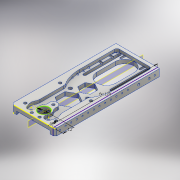
# Autodesk Inventor part: Z-head-baseplate-IKO
Saved by Autodesk Inventor 2016 (Build 200138000, 138)
## iProperties
Created: 2015-05-08
Part Number: Z-head-baseplate-IKO
Material: Aluminum 6061
Document SubType Name: Modeling
Designer: ax
Density: 2.7 g/cm^3
Appearance: Aluminum - Flat
Mass: 63.125 g
Surface Area: 166.822 cm^2
Volume: 23.3796 cm^3
Author: ax
Autodesk Inventor part; units mm, degrees
ref_plane "YZ Plane" through (0, 0, 0) normal (1, 0, 0) x (0, 1, 0)
ref_plane "XZ Plane" through (0, 0, 0) normal (0, 1, 0) x (-1, 0, 0)
ref_plane "XY Plane" through (0, 0, 0) normal (0, 0, 1) x (1, 0, 0)
sketch "Sketch1" plane through (0, 0, 0) normal (0, 0, 1) x (1, 0, 0)
  line L0 (0, 0) -> (45, 0)
  line L1 (45, 0) -> (45, 120)
  line L2 (45, 120) -> (0, 120)
  line L3 (0, 120) -> (0, 0)
  dimension "width" = 45
  dimension "height" = 120
  constraints: 8 end point, 2 parallel, 1 horizontal, 1 perpendicular
  measures "width" distance of L2.end L1.end
  measures "height" distance of L1.end L0.end
extrude "Extrusion1" add sketch "Sketch1" along normal blind 8
sketch "Sketch2" plane through (45, 0, 0) normal (1, 0, 0) x (0, 0, -1)
  line L0 (0, 0) -> (0, 120) projected
  line L1 (-8, 0) -> (-8, 120) projected
  line L2 (0, 0) -> (-8, 0)
  line L3 (-8, 0) -> (-8, 120)
  line L4 (-8, 120) -> (0, 120)
  line L5 (0, 120) -> (0, 0)
  line L6 (0, 0) -> (-8, 0) projected
  dimension "d4" = 120
  dimension "d5" = 0
  constraints: 8 end point, 2 parallel, 2 point on line, 1 horizontal, 1 perpendicular
  measures "d4" distance of L2.end L3.end
  measures "d5" distance between parallel lines of L6 L2
extrude "Extrusion2" add sketch "Sketch2" along normal blind 2.5
sketch "Sketch5" plane through (47.5, 0, 0) normal (1, 0, 0) x (0, 0, -1)
  line L0 (0, 0) -> (0, 120)
  line L1 (-8, 120) -> (-8, 0)
  line L2 (-8, 0) -> (0, 0) projected
  point P0 (-5, 12)
  point P1 (-5, 18.5)
  dimension "d11" = 6.5
  dimension "d128" = 3
  dimension "d129" = 12
  constraints: 4 end point, 1 parallel, 1 vertical
  measures "d11" distance of point (-5, 12) point (-5, 18.5)
  measures "d128" distance from line of L1 point (-5, 12)
  measures "d129" distance from line of L2 point (-5, 12)
hole "Hole1" at (47.5, 18.5, 5) at (47.5, 12, 5) direction (-1, 0, 0) diameter 1.567 depth 6.3 tip angle 118 thread size "M2x0.4" class "6H" standard "ISO Metric profile"
ref_plane "Midplane Mirror" through (22.5, 0, 0) normal (-1, 0, 0) x (0, 0, 1)
sketch "Sketch8" plane through (0, 0, 0) normal (0, 0, -1) x (-1, 0, 0)
  line L0 (-7, 116) -> (-7, 73) construction
  line L1 (-8.6, 114.4) -> (-8.6, 74.6)
  line L2 (-5.4, 74.6) -> (-5.4, 114.4)
  arc A0 (-5.4, 114.4) -> (-8.6, 114.4) centre (-7, 114.4) ccw
  arc A1 (-8.6, 74.6) -> (-5.4, 74.6) centre (-7, 74.6) ccw
  line L3 (-22.5, 120) -> (-22.5, 40) construction
  point P0 (0, 0)
  point P1 (-7, 94.5)
  dimension "d40" = 43
  dimension "d41" = 3.2
  dimension "d42" = 80
  dimension "d43" = 15.5
  constraints: 10 end point, 6 point on circle, 4 tangent, 2 centre point, 2 point on line, 2 vertical, 1 midpoint, 1 parallel
  measures "d40" distance of L0.start L0.end
  measures "d41" diameter of A1
  measures "d42" distance of L3.start L3.end
  measures "d43" distance from line of L3 point (-7, 94.5)
extrude "Extrusion3" cut sketch "Sketch8" against normal through all
sketch "Sketch9" plane through (0, 0, 8) normal (0, 0, 1) x (1, 0, 0)
  line L0 (22.5, 116) -> (22.5, 73) construction
  line L1 (11.5, 105) -> (11.5, 84)
  line L2 (33.5, 84) -> (33.5, 105)
  arc A0 (33.5, 105) -> (11.5, 105) centre (22.5, 105) ccw
  arc A1 (11.5, 84) -> (33.5, 84) centre (22.5, 84) ccw
  line L3 (0, 120) -> (0, 0) projected
  line L4 (0, 120) -> (47.5, 120) projected
  point P0 (22.5, 94.5)
  point P1 (45, 83)
  dimension "d47" = 43
  dimension "d48" = 22
  dimension "d130" = 15
  dimension "d131" = 22.5
  constraints: 8 end point, 6 point on circle, 4 tangent, 2 centre point, 2 point on line, 1 midpoint, 1 parallel, 1 vertical
  measures "d47" distance of L0.start L0.end
  measures "d48" diameter of A1
  measures "d130" distance from line of L4 A0.centre
  measures "d131" distance from line of L3 A0.centre
extrude "Extrusion4" cut sketch "Sketch9" against normal through all
sketch "Sketch10" plane through (0, 0, 0) normal (0, 0, -1) x (-1, 0, 0)
  point P0 (0, 0)
sketch "Sketch11" plane through (0, 0, 8) normal (0, 0, 1) x (1, 0, 0)
  point P0 (12.5, 52.5)
  point P1 (12.5, 7.5)
  point P2 (32.5, 52.5)
  point P3 (32.5, 7.5)
hole "Hole6" at (12.5, 52.5, 8) at (12.5, 7.5, 8) at (32.5, 52.5, 8) at (32.5, 7.5, 8) direction (0, 0, -1) diameter 4 depth 8 counterbore diameter 8 counterbore depth 3.5
sketch "Sketch13" plane through (0, 0, 8) normal (0, 0, 1) x (1, 0, 0)
  circle A0 centre (12.5, 7.5) radius 4 construction
  line L0 (12.5, 11.5) -> (32.5, 11.5) construction
  arc A1 (36.5, 7.5) -> (36.5, 7.5) centre (32.5, 7.5) ccw construction
  circle A2 centre (22.5, 12) radius 6
  circle A3 centre (22.5, 12) radius 6.55 construction
  line L1 (0, 0) -> (47.5, 0) projected
  dimension "d70" = 12
  dimension "d72" = 13.1
  dimension "d132" = 12
  constraints: 2 centre point, 2 end point, 1 coincident, 1 point on circle, 1 tangent, 1 vertical alignment, 1 other
  measures "d70" diameter of A2
  measures "d72" diameter of A3
  measures "d132" distance from line of L1 A2.centre
extrude "Extrusion5" cut sketch "Sketch13" against normal blind 4
sketch "Sketch14" plane through (22.5, 12, 4) normal (0, 0, 1) x (1, 0, 0)
  circle A0 centre (-0.0823, -0.2051) radius 5.4
  point P0 (-22.5, -12)
  dimension "d75" = 10.8
  constraints: 1 centre point
  measures "d75" diameter of A0
extrude "Extrusion6" cut sketch "Sketch14" against normal through all
sketch "Sketch15" plane through (0, 0, 0) normal (0, 0, -1) x (-1, 0, 0)
  point P0 (-27, 2.75)
  point P1 (-22.5, 23)
  point P2 (-18, 2.75)
hole "Hole9" at (27, 2.75, 0) at (22.5, 23, 0) at (18, 2.75, 0) direction (0, 0, 1) diameter 3.1 depth 8 counterbore diameter 6 counterbore depth 2.3
sketch "Sketch17" plane through (0, 0, 0) normal (0, 0, -1) x (-1, 0, 0)
  point P0 (-40.2, 48.5)
  point P1 (-40.2, 8.5)
hole "Hole12" at (40.2, 48.5, 0) at (40.2, 8.5, 0) direction (0, 0, 1) diameter 3.2 depth 8 counterbore diameter 6.5 counterbore depth 3.4
sketch "Sketch18" plane through (0, 0, 0) normal (-1, 0, 0) x (0, 0, 1)
  line L0 (0, 120) -> (0, 0) projected
  line L1 (0, 0) -> (8, 0)
  line L2 (8, 0) -> (8, 120)
  line L3 (8, 120) -> (0, 120)
  line L4 (0, 120) -> (0, 0)
  constraints: 8 end point, 2 parallel, 1 horizontal, 1 perpendicular
extrude "Extrusion7" add sketch "Sketch18" along normal blind 2.5
sketch "Sketch19" plane through (47.5, 120, 8) normal (0, 1, 0) x (1, 0, 0)
  line L0 (0, 8) -> (0, 0) projected
  line L1 (-50, 0) -> (0, 0) projected
  point P0 (-47.5, 8)
  point P1 (-4, 4)
  point P2 (-14, 4)
  dimension "d133" = 4
  dimension "d134" = 4
  dimension "d135" = 10
  dimension "d136" = 0
  measures "d133" distance from line of L0 point (-4, 4)
  measures "d134" distance from line of L1 point (-4, 4)
  measures "d135" distance of point (-14, 4) point (-4, 4)
  measures "d136" vertical distance of point (-14, 4) point (-4, 4)
hole "Hole14" at (33.5, 120, 4) at (43.5, 120, 4) direction (0, -1, 0) diameter 2.459 depth 8.8 tip angle 118 thread size "M3x0.5" class "6H" standard "ISO Metric profile"
sketch "Sketch20" plane through (47.5, 0, 0) normal (1, 0, 0) x (0, 0, -1)
  line L0 (0, 120) -> (-8, 120) projected
  line L1 (0, 0) -> (0, 120) projected
  point P0 (-4, 108)
  point P1 (-4, 96)
  dimension "d144" = 12
  dimension "d145" = 12
  dimension "d146" = 4
  dimension "d147" = 4
  measures "d144" distance from line of L0 point (-4, 108)
  measures "d145" distance of point (-4, 108) point (-4, 96)
  measures "d146" distance from line of L1 point (-4, 108)
  measures "d147" distance from line of L1 point (-4, 96)
hole "Hole15" at (47.5, 108, 4) at (47.5, 96, 4) direction (-1, 0, 0) diameter 2.459 depth 8.8 tip angle 118 thread size "M3x0.5" class "6H" standard "ISO Metric profile"
mirror "Mirror1" about plane through (22.5, 0, 0) normal (-1, 0, 0) of "Extrusion3"
mirror "Mirror2" about plane through (22.5, 0, 0) normal (-1, 0, 0) of "Hole15", "Hole14", "Hole12"
sketch "Sketch22" plane through (0, 0, 8) normal (0, 0, 1) x (1, 0, 0)
  circle A0 centre (40.2, 48.5) radius 1.6
  circle A1 centre (40.2, 8.5) radius 1.6
  circle A2 centre (22.5, 12) radius 6
  circle A3 centre (27, 2.75) radius 1.55
  circle A4 centre (22.5, 23) radius 1.55
  arc A5 (27.05, 23) -> (22.5, 27.55) centre (22.5, 23) ccw
  circle A6 centre (32.5, 7.5) radius 4
  circle A7 centre (12.5, 7.5) radius 4
  line L0 (22.5, 27.55) -> (22.5, 69.55)
  arc A8 (11.5, 84) -> (33.5, 84) centre (22.5, 84) ccw
  line L1 (22.5, 69.55) -> (22.5, 76.0732)
  line L2 (36.4, 74.6) -> (36.4, 114.4) construction
  arc A9 (36.4, 74.6) -> (39.6, 74.6) centre (38, 74.6) ccw construction
  line L3 (39.6, 114.4) -> (39.6, 74.6) construction
  line L4 (47.5, 0) -> (-2.5, 0)
  line L5 (47.5, 120) -> (47.5, 0)
  line L6 (26.4052, 20.3293) -> (27.05, 23) construction
  spline S0 degree 3 poles (29.1413, 16) (27.3688, 17.8667) (26.4052, 20.3293) (27.05, 23) knots 0 0 0 0 1 1 1 1
  line L7 (29.1413, 16) -> (27.3688, 17.8667) construction
  line L8 (27.3688, 17.8667) -> (26.4052, 20.3293) construction
  line L9 (29.1413, 16) -> (29.9178, 12.7953) construction
  line L10 (29.9178, 12.7953) -> (29.1413, 9.6723) construction
  spline S1 degree 2 poles (29.1413, 16) (29.9178, 12.7953) (29.1413, 9.6723) knots 1 1 1 2 2 2
  line L11 (35.653, 47.8037) -> (35.653, 20.8037)
  line L12 (35.653, 20.8037) -> (35.653, 16.2873) construction
  line L13 (35.653, 16.2873) -> (38.534, 14.0658) construction
  line L14 (38.534, 14.0658) -> (38.534, 14.1201) construction
  line L15 (38.534, 14.1201) -> (36.2949, 6.2356) construction
  spline S2 degree 4 poles (35.653, 20.8037) (35.653, 16.2873) (38.534, 14.0658) (38.534, 14.1201) (36.2949, 6.2356) knots 1 1 1 1 1 2 2 2 2 2
  line L16 (22.5, 76.0732) -> (22.5, 116.2002)
  line L17 (22.5, 116.2002) -> (29.1413, 116.2002)
  line L18 (29.1413, 116.2002) -> (39.5413, 116.2002)
  line L19 (42.6413, 113.1002) -> (42.6413, 73.0462)
  arc A10 (36.4, 51.0923) -> (35.653, 47.8037) centre (40.2, 48.5) ccw
  line L20 (42.6413, 73.0462) -> (42.6413, 67.447) construction
  line L21 (42.6413, 67.447) -> (41.0617, 57.6095) construction
  line L22 (41.0617, 57.6095) -> (36.4, 51.0923) construction
  spline S3 degree 3 poles (42.6413, 73.0462) (42.6413, 67.447) (41.0617, 57.6095) (36.4, 51.0923) knots 1 1 1 1 2 2 2 2
  arc A11 (42.6413, 113.1002) -> (39.5413, 116.2002) centre (39.5413, 113.1002) ccw
  point P0 (0, 0)
  point P1 (42.6413, 116.2002)
  dimension "d156" = 3
  dimension "d159" = 42
  dimension "d165" = 27
  dimension "d190" = 25
  dimension "d191" = 13.5
  dimension "d192" = 3.1
  constraints: 14 end point, 9 point on circle, 6 vertical, 5 point on line, 3 centre point, 2 tangent, 1 perpendicular, 12 other
  measures "d156" radial gap between concentric circles of A4 A5
  measures "d159" distance of L0.start L0.end
  measures "d165" distance of L11.start L11.end
  measures "d190" distance between parallel lines of L5 L0
  measures "d191" distance of L17.end point (42.641, 116.2)
  measures "d192" radius of A11
extrude "Extrusion8" cut sketch "Sketch22" against normal blind 3.5 contours A5 L0 L1 L16 L17 L18 A11 L19 S3 A10 L11 S2 A6 S1 S0 | A6 S2 picked at (33.507, 9.2958)
sketch "Sketch23" plane through (0, 0, 0) normal (0, 0, -1) x (-1, 0, 0)
  circle A0 centre (-40.2, 8.5) radius 3.25 projected
  circle A1 centre (-40.2, 48.5) radius 3.25 projected
  line L0 (-36.95, 48.5) -> (-36.95, 8.5)
  circle A2 centre (-40.2, 48.5) radius 3.25 projected
  line L1 (-43.448, 48.6132) -> (-43.448, 8.6132)
  circle A3 centre (-40.2, 8.5) radius 3.25 projected
  circle A4 centre (-32.5, 7.5) radius 2 projected
  line L2 (-36.95, 8.5) -> (-36.95, 4.0252) construction
  spline S0 degree 3 poles (-36.95, 8.5) (-36.95, 4.0252) (-32.87, 3.6199) (-30.3103, 4.392) knots 1 1 1 1 1.838828 1.838828 1.838828 1.838828
  line L3 (-19.199, 0) -> (-25.801, 0) projected
  line L4 (-22.5, 0) -> (-41.7217, 0)
  line L5 (-43.448, 8.6132) -> (-43.448, 5.109)
  line L6 (-41.7217, 1.34) -> (-41.7217, 0)
  line L7 (-41.7217, 0) -> (-22.5, 0)
  line L8 (-22.5, 0) -> (-41.7217, 0)
  line L9 (-22.5, 0) -> (-22.5, 5.109)
  line L10 (-22.5, 5.109) -> (-23.3472, 5.109)
  line L11 (-23.3472, 5.109) -> (-24.493, 5.109) construction
  line L12 (-24.493, 5.109) -> (-27.4923, 6.6797) construction
  line L13 (-27.4923, 6.6797) -> (-28.734, 5.6052) construction
  line L14 (-28.734, 5.6052) -> (-30.3103, 4.392) construction
  spline S1 degree 4 poles (-23.3472, 5.109) (-24.493, 5.109) (-27.4923, 6.6797) (-28.734, 5.6052) (-30.3103, 4.392) knots 1 1 1 1 1 2 2 2 2 2
  line L15 (-36.95, 4.0252) -> (-32.87, 3.6199) construction
  line L16 (-32.87, 3.6199) -> (-30.3103, 4.392) construction
  arc A5 (-41.7217, 1.34) -> (-42.4013, 2.8306) centre (-43.6962, 1.34) ccw
  arc A6 (-43.448, 5.109) -> (-42.4013, 2.8306) centre (-40.4451, 5.109) ccw
  dimension "d166" = 40
  constraints: 18 end point, 6 point on circle, 6 vertical, 2 centre point, 2 horizontal, 2 tangent, 1 collinear, 1 horizontal alignment, 1 midpoint, 1 perpendicular, 11 other
  measures "d166" distance of L1.start L1.end
extrude "Extrusion9" cut sketch "Sketch23" against normal blind 3.5 contours S0 S1 L10 L9 L3 L4 L6 A5 A6 L5 A0 | A0 L1 A1 L0 | A1
mirror "Mirror3" about plane through (22.5, 0, 0) normal (-1, 0, 0) of "Extrusion8", "Extrusion9"
chamfer "Chamfer1" distance 2 angle 45 2 edges at (47.5, 0, 4) (-2.5, 0, 4)
chamfer "Chamfer2" distance 0.2 angle 45 2 edges at (47.5, 120, 4) (-2.5, 120, 4)
sketch "Sketch24" plane through (7, 114.4, 4.5) normal (0, 0, 1) x (1, 0, 0)
  line L0 (5.5407, -68.15) -> (15.5, -62.4)
  line L1 (15.5, -62.4) -> (25.4593, -68.15)
  line L2 (25.4593, -68.15) -> (25.4593, -79.65)
  line L3 (25.4593, -79.65) -> (15.5, -85.4)
  line L4 (15.5, -85.4) -> (5.5407, -79.65)
  line L5 (5.5407, -79.65) -> (5.5407, -68.15)
  line L6 (15.5, -138.4) -> (15.5, 29.6) projected
  arc A0 (20.05, -91.4) -> (10.95, -91.4) centre (15.5, -91.4) ccw projected
  line L7 (8.1388, -47.65) -> (15.5, -43.4)
  line L8 (15.5, -43.4) -> (22.8612, -47.65)
  line L9 (22.8612, -47.65) -> (22.8612, -56.15)
  line L10 (22.8612, -56.15) -> (15.5, -60.4)
  line L11 (15.5, -60.4) -> (8.1388, -56.15)
  line L12 (8.1388, -56.15) -> (8.1388, -47.65)
  point P0 (-7, -114.4)
  point P1 (15.5, -73.9)
  point P2 (15.5, -51.9)
  dimension "d193" = 0
  dimension "d194" = 6
  dimension "d195" = 11.5
  dimension "d199" = 8.5
  dimension "d200" = 0
  dimension "d201" = 2
  constraints: 24 end point, 1 parallel, 26 other
  measures "d193" distance from line of L6 point (15.5, -73.9)
  measures "d194" distance of A0.centre L3.end
  measures "d195" distance of L4.end L0.start
  measures "d199" distance of L11.end L7.start
  measures "d200" distance from line of L6 point (15.5, -51.9)
  measures "d201" distance of L0.end L10.end
extrude "Extrusion10" cut sketch "Sketch24" against normal through all
fillet "Fillet2" radius 1 12 edges at (12.5407, 46.25, 2.25) (12.5407, 34.75, 2.25) (22.5, 29, 2.25) (32.4593, 34.75, 2.25) (32.4593, 46.25, 2.25) (22.5, 52, 2.25) (15.1388, 58.25, 2.25) (15.1388, 66.75, 2.25) (22.5, 71, 2.25) (29.8612, 66.75, 2.25) (29.8612, 58.25, 2.25) (22.5, 54, 2.25)
sketch "Sketch27" plane through (47.5, 0, 0) normal (1, 0, 0) x (0, 0, -1)
  line L0 (-8, 0) -> (0, 0) projected
  line L1 (0, 2) -> (0, 119.8) projected
  line L2 (0, 120) -> (-8, 120) projected
  point P0 (-4, 5.5)
  point P1 (-4, 114.5)
  dimension "d216" = 5.5
  dimension "d217" = 4
  dimension "d218" = 4
  dimension "d219" = 5.5
  measures "d216" distance from line of L0 point (-4, 5.5)
  measures "d217" distance from line of L1 point (-4, 5.5)
  measures "d218" distance from line of L1 point (-4, 114.5)
  measures "d219" distance from line of L2 point (-4, 114.5)
hole "Hole20" at (47.5, 5.5, 4) at (47.5, 114.5, 4) direction (-1, 0, 0) diameter 1.567 depth 6.3 tip angle 118 thread size "M2x0.4" class "6H" standard "ISO Metric profile"
mirror "Mirror4" about plane through (22.5, 0, 0) normal (-1, 0, 0) of "Hole20"
pattern_linear "Rectangular Pattern3" count 6 spacing 13 along (0, 1, 0) of "Hole1"
mirror "Mirror5" about plane through (22.5, 0, 0) normal (-1, 0, 0) of "Hole1", "Rectangular Pattern3"
sketch "Sketch25" plane through (-2.3, 120, 8) normal (0, 1, 0) x (1, 0, 0)
  point P0 (13.8, 4)
  point P1 (35.8, 4)
  point P2 (45.8, 4)
  point P3 (3.8, 4)
sketch "Sketch26" plane through (-2.5, 0, 0) normal (-1, 0, 0) x (0, 0, 1)
  point P0 (4, 108)
  point P1 (4, 96)
equation "\"d4\" = height"
equation "\"d131\" = 0.5 * width"
equation "\"d147\" = d146"
equation "\"d25\" = -0.5 * width"
body "Solid1"
